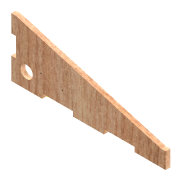
# Autodesk Inventor part: zijkant elektrobox voor knop
Saved by Autodesk Inventor 2020.3 (Build 243373000, 373)
## iProperties
Created: 2020-11-26
Part Number: zijkant elektrobox voor knop
Material: Wood (Birch)
Document SubType Name: Sheet Metal
Designer: Svend
Density: 0.55 g/cm^3
Sheet Metal Rule: Default_mm
Appearance: Birch - Natural Polished
Author: Svend
Autodesk Inventor part; units mm, degrees
ref_plane "YZ Plane" through (0, 0, 0) normal (1, 0, 0) x (0, 1, 0)
ref_plane "XZ Plane" through (0, 0, 0) normal (0, 1, 0) x (-1, 0, 0)
ref_plane "XY Plane" through (0, 0, 0) normal (0, 0, 1) x (1, 0, 0)
ref_plane "Work Plane1" through (0, 0, 0) normal (0, 0, 1) x (1, 0, 0)
sketch "Sketch1" plane through (0, 0, 0) normal (0, 0, 1) x (1, 0, 0)
  line L0 (0, 6) -> (40, 6)
  line L1 (0, 0) -> (0, 6)
  line L2 (40, 0) -> (0, 0)
  line L3 (40, 0) -> (40, 6)
  line L4 (80, 0) -> (80, 6)
  line L5 (80, 6) -> (40, 6)
  line L6 (40, 6) -> (40, 0)
  line L7 (40, 0) -> (80, 0)
  line L8 (80, 6) -> (120, 6)
  line L9 (80, 0) -> (80, 6)
  line L10 (120, 0) -> (80, 0)
  line L11 (120, 0) -> (120, 6)
  line L12 (160, 0) -> (160, 6)
  line L13 (160, 6) -> (120, 6)
  line L14 (120, 6) -> (120, 0)
  line L15 (120, 0) -> (160, 0)
  line L16 (160, 6) -> (200, 6)
  line L17 (160, 0) -> (160, 6)
  line L18 (200, 0) -> (160, 0)
  line L19 (200, 6) -> (200, 0)
  line L20 (200, 6) -> (200, 21)
  line L21 (194, 21) -> (200, 21)
  line L22 (194, 21) -> (194, 6)
  line L23 (194, 6) -> (200, 6)
  line L24 (6, 28.5) -> (0, 28.5)
  line L25 (0, 28.5) -> (0, 6)
  line L26 (6, 6) -> (0, 6)
  line L27 (6, 6) -> (6, 28.5)
  line L28 (0, 53.5) -> (0, 28.5)
  line L29 (6, 28.5) -> (0, 28.5)
  line L30 (6, 28.5) -> (6, 53.5)
  line L31 (6, 53.5) -> (0, 53.5)
  line L32 (6, 53.5) -> (0, 53.5)
  line L33 (6, 53.5) -> (6, 76)
  line L34 (6, 76) -> (0, 76)
  line L35 (0, 76) -> (0, 53.5)
  line L36 (6, 76) -> (194, 21)
extrude "Plate1" add sketch "Sketch1" along normal blind 6 contours L25 L24 L27 L0 | L0 L3 L2 L1 | L27 L30 L33 L36 L22 L16 L13 L8 L5 L0 | L35 L34 L33 L31 | L8 L11 L10 L4 | L16 L19 L18 L12 | L21 L20 L16 L22
sketch "Sketch2" plane through (0, 0, 6) normal (0, 0, 1) x (1, 0, 0)
  line L0 (0, 0) -> (0, 28.5) projected
  line L1 (40, 0) -> (0, 0) projected
  line L2 (40, 6) -> (40, 0) projected
  line L3 (80, 6) -> (40, 6) projected
  line L4 (80, 0) -> (80, 6) projected
  line L5 (120, 0) -> (80, 0) projected
  line L6 (120, 6) -> (120, 0) projected
  line L7 (160, 6) -> (120, 6) projected
  line L8 (160, 0) -> (160, 6) projected
  line L9 (200, 0) -> (160, 0) projected
  line L10 (200, 21) -> (200, 0) projected
  line L11 (194, 21) -> (200, 21) projected
  line L12 (6, 76) -> (194, 21) projected
  line L13 (0, 76) -> (6, 76) projected
  line L14 (0, 53.5) -> (0, 76) projected
  line L15 (6, 53.5) -> (0, 53.5) projected
  line L16 (6, 28.5) -> (6, 53.5) projected
  line L17 (0, 28.5) -> (6, 28.5) projected
  circle A0 centre (20, 20) radius 8
  point P0 (0, 0)
  point P1 (20, 0)
  dimension "d1" = 16
  dimension "d2" = 20
  constraints: 1 centre point, 1 midpoint, 1 vertical alignment
  measures "d1" diameter of A0
  measures "d2" distance from line of L1 A0.centre
extrude "Cut1" cut sketch "Sketch2" against normal blind 6 contours A0
equation "\"d3\" = Thickness"
equation "\"d0\" = Thickness"
equation "\"BendRadius\" = Thickness"
equation "\"BendReliefWidth\" = Thickness"
equation "\"BendReliefDepth\" = 0.5 * Thickness"
equation "\"CornerReliefSize\" = 4 * Thickness"
equation "\"MinimumRemnant\" = 2 * Thickness"
equation "\"TransitionRadius\" = BendRadius"
equation "\"JacobiRadiusSize\" = BendRadius"
equation "\"GapSize\" = Thickness"
equation "\"Thickness\" = 6"
body "Solid1"
